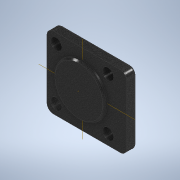
# Autodesk Inventor part: cylinder head
Saved by Autodesk Inventor 2021.1 (Build 251245000, 245)
## iProperties
Created: 2020-08-30
Part Number: cylinder head
Material: Aluminum 6061
Document SubType Name: Sheet Metal
Designer: Vamshi
Mass: 620.061 g
Surface Area: 377.616 cm^2
Volume: 229.652 cm^3
Density: 2.7 g/cm^3
Sheet Metal Rule: Default
Appearance: Black Cast
Author: Vamshi
Autodesk Inventor part; units mm, degrees
ref_plane "YZ Plane" through (0, 0, 0) normal (1, 0, 0) x (0, 1, 0)
ref_plane "XZ Plane" through (0, 0, 0) normal (0, 1, 0) x (-1, 0, 0)
ref_plane "XY Plane" through (0, 0, 0) normal (0, 0, 1) x (1, 0, 0)
sketch "Sketch1" plane through (0, 0, 0) normal (0, 0, 1) x (1, 0, 0)
  line L0 (-45.72, 57.15) -> (60.96, 57.15)
  line L1 (71.12, 46.99) -> (71.12, -46.99)
  line L2 (60.96, -57.15) -> (-45.72, -57.15)
  line L3 (-55.88, -46.99) -> (-55.88, 46.99)
  line L4 (-85.7425, 0) -> (99.7187, 0) projected
  line L5 (0, -82.9559) -> (0, 82.9559) projected
  circle A0 centre (0, 0) radius 40.64
  circle A1 centre (0, 0) radius 58.42 construction
  line L6 (0, 0) -> (-59.2481, 59.2481) construction
  circle A2 centre (-41.3092, 41.3092) radius 8.89
  circle A3 centre (-41.3092, -41.3092) radius 8.89
  circle A4 centre (41.3092, -41.3092) radius 8.89
  circle A5 centre (41.3092, 41.3092) radius 8.89
  arc A6 (-45.72, 57.15) -> (-55.88, 46.99) centre (-45.72, 46.99) ccw
  arc A7 (71.12, 46.99) -> (60.96, 57.15) centre (60.96, 46.99) ccw
  arc A8 (60.96, -57.15) -> (71.12, -46.99) centre (60.96, -46.99) ccw
  arc A9 (-55.88, -46.99) -> (-45.72, -57.15) centre (-45.72, -46.99) ccw
  point P0 (71.12, -57.15)
  point P1 (71.12, 57.15)
  point P2 (-55.88, -57.15)
  point P3 (71.12, 0)
  dimension "d4" = 116.84
  dimension "d0" = 127
  dimension "d1" = 114.3
  dimension "d2" = 55.88
  dimension "d3" = 81.28
  dimension "d5" = 45
  dimension "d6" = 17.78
  dimension "d9" = 360
  dimension "d11" = 10.16
  dimension "d12" = 59.2481
  constraints: 10 end point, 9 centre point, 8 point on circle, 8 point on line, 8 tangent, 3 equal radius, 2 coincident, 2 parallel, 1 horizontal, 1 midpoint, 1 perpendicular, 12 other
  measures "d0" distance of point (71.12, -57.15) point (-55.88, -57.15)
  measures "d1" distance of point (71.12, 57.15) point (71.12, -57.15)
  measures "d2" distance between parallel lines of L5 L3
  measures "d3" diameter of A0
  measures "d5" angle of L4 L6
  measures "d6" diameter of A2
  measures "d11" radius of A6
  measures "d12" distance from line of L6.end L5
extrude "Extrusion1" add sketch "Sketch1" against normal blind 15.24
extrude "Extrusion2" add sketch "Sketch1" along normal blind 5.08 contours A0 L4 L5 | L5 L4 A0 | L5 A0 L4 | L4 A0 L5
chamfer "Chamfer1" distance 2.54 angle 45 1 edges at (-40.64, 0, 5.08) measured on face at (4.2922, -0.5549, 5.08)
fillet "Fillet1" radius 2.54 8 edges at (68.1442, 54.1742, -15.24) (71.12, 0, -15.24) (68.1442, -54.1742, -15.24) (7.62, -57.15, -15.24) (-52.9042, -54.1742, -15.24) (-55.88, 0, -15.24) (-52.9042, 54.1742, -15.24) (7.62, 57.15, -15.24)
equation "\"BendRadius\" = Thickness"
equation "\"BendReliefWidth\" = Thickness"
equation "\"BendReliefDepth\" = 0.5 * Thickness"
equation "\"CornerReliefSize\" = 4 * Thickness"
equation "\"MinimumRemnant\" = 2 * Thickness"
equation "\"TransitionRadius\" = BendRadius"
equation "\"JacobiRadiusSize\" = BendRadius"
equation "\"GapSize\" = Thickness"
equation "\"Thickness\" = 3.048"
body "Solid1"
